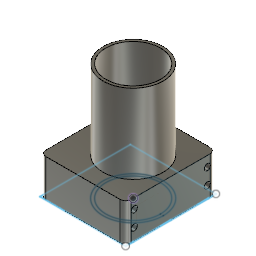
soporte de ruedas 16-5QWqw v1 (Autodesk Fusion 360 design; units mm, degrees)
Autodesk Fusion 360 part; units mm, degrees
sketch "Boceto8" plane through (0, 0, 0) normal (0, 0, 1) x (1, 0, 0)
sketch "Boceto9" plane through (0, 0, 0) normal (0, 0, 1) x (1, 0, 0)
  circle A0 centre (0, 0) radius 14.5
  line L0 (20, 0) -> (20, 20)
  line L1 (20, 0) -> (20, -20)
  circle A1 centre (0, 0) radius 16
  line L2 (20, 20) -> (20, 24)
  line L3 (20, -20) -> (20, -24)
  line L4 (20, -20) -> (20, -24)
  line L5 (20, 0) -> (20, 20)
  line L6 (20, 0) -> (20, -20)
  circle A2 centre (0, 0) radius 16
  circle A3 centre (0, 0) radius 14.5
  line L7 (20, 20) -> (20, 24)
  line L8 (-25.5, 24) -> (-25.5, -24)
  line L9 (-25.5, 24) -> (20, 24)
  line L10 (20, -24) -> (-25.5, -24)
  dimension "d26" = 29
  dimension "d27" = 20
  dimension "d36" = 32
  dimension "d63" = 29
  dimension "d64" = 20
  dimension "d65" = 32
  constraint coincident A0.centre A1.centre
  constraint perpendicular L2 L9
  constraint perpendicular L8 L10
  measures "d26" diameter of A0
  measures "d27" distance of A0.centre L0.start
  measures "d36" diameter of A1
  measures "d63" diameter of A3
  measures "d64" distance of L0.start A0.centre
  measures "d65" diameter of A2
extrude "Extruir8" add sketch "Boceto9" along normal blind 62 contours A1 A2
extrude "Extruir10" add sketch "Boceto9" along normal blind 20 contours L0 L1 L2 L3 L4 L5 L6 L7 L8 L9 L10
fillet "Empalme3" radius 3 4 edges at (-25.5, -24, 10) (-25.5, 24, 10) (20, 24, 10) (20, -24, 10)
hole "Agujero6" at (20, 19.4786, 14.6367) direction (-1, 0, 0) diameter 3.25 depth 80 tip angle 118
hole "Agujero7" at (20, 19.4389, 6.2793) direction (-1, 0, 0) diameter 3.25 depth 80 tip angle 118
sketch "Boceto11" plane through (20, 0, 0) normal (1, 0, 0) x (0, 1, 0)
  arc A0 (21, 6.7303) -> (21, 5.8282) centre (19.4389, 6.2793) ccw
  line L0 (21, 6.7303) -> (21, 14.0658)
  arc A1 (21, 15.2076) -> (21, 14.0658) centre (19.4786, 14.6367) ccw
  line L1 (21, 15.2076) -> (21, 20)
  line L2 (21, 20) -> (-21, 20)
  line L3 (-21, 20) -> (-21, 0)
  line L4 (-21, 0) -> (21, 0)
  line L5 (21, 0) -> (21, 5.8282)
hole "Agujero8" at (20, -19.3772, 14.6266) direction (-1, 0, 0) diameter 3.25 depth 80 tip angle 118
hole "Agujero9" at (20, -19.413, 6.2987) direction (-1, 0, 0) diameter 3.25 depth 80 tip angle 118
extrude "Extruir9" [suppressed]
